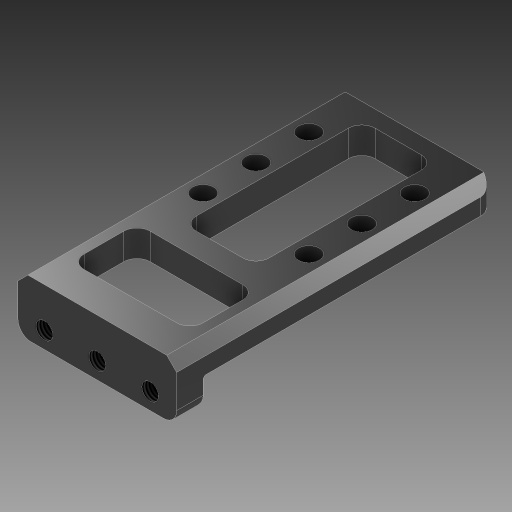
# Autodesk Inventor part: 254 Cross Block
Saved by Autodesk Inventor 2024 (Build 280153000, 153)
## iProperties
Created: 2023-07-01
Part Number: 254 Cross Block
Material: Aluminum 6061
Document SubType Name: Modeling
Designer: Max Boord
Mass: 30.2094 g
Surface Area: 70.2847 cm^2
Volume: 11.1887 cm^3
Density: 2.7 g/cm^3
Appearance: Glossy - Black
Author: Max Boord
Autodesk Inventor part; units mm, degrees
ref_plane "YZ Plane" through (0, 0, 0) normal (1, 0, 0) x (0, 1, 0)
ref_plane "XZ Plane" through (0, 0, 0) normal (0, 1, 0) x (-1, 0, 0)
ref_plane "XY Plane" through (0, 0, 0) normal (0, 0, 1) x (1, 0, 0)
sketch "Sketch1" plane through (0, 0, 0) normal (0, 1, 0) x (-1, 0, 0)
  line L0 (-19.05, -38.1) -> (19.05, -38.1)
  line L1 (19.05, -38.1) -> (19.05, 38.1)
  line L2 (19.05, 38.1) -> (-19.05, 38.1)
  line L3 (-19.05, 38.1) -> (-19.05, -38.1)
  line L4 (-19.05, -38.1) -> (19.05, 38.1) construction
  line L5 (19.05, -38.1) -> (-19.05, 38.1) construction
  circle A0 centre (12.7, -25.4) radius 2.4892
  circle A1 centre (12.7, -12.7) radius 2.4892
  circle A2 centre (12.7, 0) radius 2.4892
  circle A3 centre (-12.7, -25.4) radius 2.4892
  circle A4 centre (-12.7, -12.7) radius 2.4892
  circle A5 centre (-12.7, 0) radius 2.4892
  line L6 (-12.7, -25.4) -> (12.7, -25.4) construction
  line L7 (-19.05, 12.7) -> (19.05, 12.7)
  line L8 (-19.05, 31.75) -> (19.05, 31.75)
  line L9 (-5.5562, 8.7313) -> (5.5563, 8.7313)
  line L10 (8.7313, 5.5563) -> (8.7313, -30.9563)
  line L11 (5.5563, -34.1313) -> (-5.5562, -34.1313)
  line L12 (-8.7312, -30.9563) -> (-8.7312, 5.5563)
  line L13 (-8.7313, 8.7313) -> (8.7313, -34.1313) construction
  line L14 (8.7313, 8.7313) -> (-8.7312, -34.1313) construction
  line L15 (-11.1125, 30.1625) -> (11.1125, 30.1625)
  line L16 (14.2875, 26.9875) -> (14.2875, 17.4625)
  line L17 (11.1125, 14.2875) -> (-11.1125, 14.2875)
  line L18 (-14.2875, 17.4625) -> (-14.2875, 26.9875)
  line L19 (-14.2875, 30.1625) -> (14.2875, 14.2875) construction
  line L20 (14.2875, 30.1625) -> (-14.2875, 14.2875) construction
  line L21 (-12.7, -25.4) -> (-12.7, -12.7)
  arc A6 (-8.7312, -30.9563) -> (-5.5562, -34.1313) centre (-5.5562, -30.9563) ccw
  arc A7 (5.5563, -34.1313) -> (8.7313, -30.9563) centre (5.5563, -30.9563) ccw
  arc A8 (8.7313, 5.5563) -> (5.5563, 8.7313) centre (5.5563, 5.5563) ccw
  arc A9 (-5.5562, 8.7313) -> (-8.7312, 5.5563) centre (-5.5562, 5.5563) ccw
  arc A10 (-14.2875, 17.4625) -> (-11.1125, 14.2875) centre (-11.1125, 17.4625) ccw
  arc A11 (11.1125, 14.2875) -> (14.2875, 17.4625) centre (11.1125, 17.4625) ccw
  arc A12 (14.2875, 26.9875) -> (11.1125, 30.1625) centre (11.1125, 26.9875) ccw
  arc A13 (-11.1125, 30.1625) -> (-14.2875, 26.9875) centre (-11.1125, 26.9875) ccw
  line L22 (-16.6687, -38.1) -> (-16.6687, 38.1)
  point P0 (0, 0)
  point P1 (0, -25.4)
  point P2 (0, -38.1)
  point P3 (0, -12.7)
  point P4 (0, 22.225)
  dimension "d0" = 38.1
  dimension "d1" = 76.2
  dimension "d2" = 4.9784
  dimension "d5" = 12.7
  dimension "d8" = 25.4
  dimension "d11" = 12.7
  dimension "d12" = 50.8
  dimension "d13" = 25.4
  dimension "d14" = 6.35
  dimension "d15" = 3.9688
  dimension "d17" = 4.7625
  dimension "d18" = 3.175
  dimension "d19" = 1.5875
  dimension "d20" = 1.5875
  dimension "d61" = 2.3813
  dimension "d62" = 7.9375
  constraints: 46 end point, 22 point on line, 16 point on circle, 16 tangent, 14 centre point, 8 midpoint, 7 equal radius, 6 parallel, 6 perpendicular, 5 horizontal, 3 vertical alignment, 2 vertical, 1 horizontal alignment, 11 other
  measures "d0" distance of L2.end L1.end
  measures "d1" distance of L1.end L0.end
  measures "d2" diameter of A0
  measures "d5" distance of L6.end A1.centre
  measures "d8" distance of L6.end L6.start
  measures "d11" distance from line of L0 L6.start
  measures "d12" distance between parallel lines of L0 L7
  measures "d13" distance between parallel lines of L2 L7
  measures "d14" distance between parallel lines of L2 L8
  measures "d15" distance between parallel lines of L0 L11
  measures "d17" distance between parallel lines of L3 L18
  measures "d18" radius of A6
  measures "d19" distance between parallel lines of L7 L17
  measures "d20" distance between parallel lines of L8 L15
  measures "d61" distance between parallel lines of L3 L22
  measures "d62" diameter of L22 L21
extrude "Extrusion1" add sketch "Sketch1" along normal blind 6.35
sketch "Sketch3" plane through (-19.05, 0, 38.1) normal (0, 0, 1) x (1, 0, 0)
  line L0 (0, 0) -> (38.1, 0) projected
  line L1 (38.1, 0) -> (38.1, 6.35) projected
  line L2 (0, 6.35) -> (38.1, 6.35) projected
  line L3 (0, 0) -> (0, 6.35) projected
  line L4 (34.925, -7.1438) -> (3.175, -7.1438)
  line L5 (0, -3.9688) -> (0, 0)
  line L6 (38.1, 0) -> (38.1, -3.9688)
  circle A0 centre (31.75, -3.175) radius 1.27
  circle A1 centre (19.05, -3.175) radius 1.27
  circle A2 centre (6.35, -3.175) radius 1.27
  arc A3 (34.925, -7.1438) -> (38.1, -3.9688) centre (34.925, -3.9688) ccw
  arc A4 (0, -3.9688) -> (3.175, -7.1438) centre (3.175, -3.9688) ccw
  point P0 (19.05, 0)
  point P1 (19.05, 6.35)
  dimension "d46" = 2.54
  dimension "d49" = 12.7
  dimension "d54" = 9.525
  dimension "d55" = 3.9688
  dimension "d56" = 13.4938
  dimension "d57" = 3.175
  constraints: 6 end point, 5 centre point, 4 point on circle, 4 tangent, 2 horizontal, 1 equal radius, 1 midpoint, 1 parallel, 1 perpendicular, 1 vertical alignment, 4 other
  measures "d46" diameter of A0
  measures "d49" distance of A0.centre A1.centre
  measures "d54" distance from line of L2 A1.centre
  measures "d55" distance from line of L4 A1.centre
  measures "d56" distance between parallel lines of L2 L4
  measures "d57" radius of A3
extrude "Extrusion3" add sketch "Sketch3" against normal blind 6.35 contours L0 L6 A3 L4 A4 L5
sketch "Sketch4" plane through (-19.05, 6.35, 38.1) normal (0, 0, 1) x (1, 0, 0)
  circle A0 centre (31.75, -9.525) radius 1.27 projected
  circle A1 centre (19.05, -9.525) radius 1.27 projected
  circle A2 centre (6.35, -9.525) radius 1.27 projected
  point P0 (19.05, -6.35)
  point P1 (31.2738, -6.35)
  point P2 (33.8137, -6.35)
  point P3 (18.5737, -6.35)
  point P4 (21.1137, -6.35)
  point P5 (5.8737, -6.35)
  point P6 (8.4137, -6.35)
  constraints: 3 coincident, 3 other
hole "Hole2" at (12.7, -3.175, 38.1) at (0, -3.175, 38.1) at (-12.7, -3.175, 38.1) direction (0, 0, -1) diameter 3.9624 depth 6.35 thread size "10-32 UNF" class "2B" standard "ANSI Unified Screw Threads"
chamfer "Chamfer2" distance 2.3813 angle 45 2 edges at (19.05, 6.35, 0) (-19.05, 6.35, 0)
fillet "Fillet1" radius 3.175 2 edges at (19.05, 1.9844, -38.1) (-19.05, 1.9844, -38.1)
fillet "Fillet3" radius 0.762 1 edges at (0, 0, 31.75)
equation "\"d20\" = d19"
equation "\"d70\" = d61"
body "Solid1"
